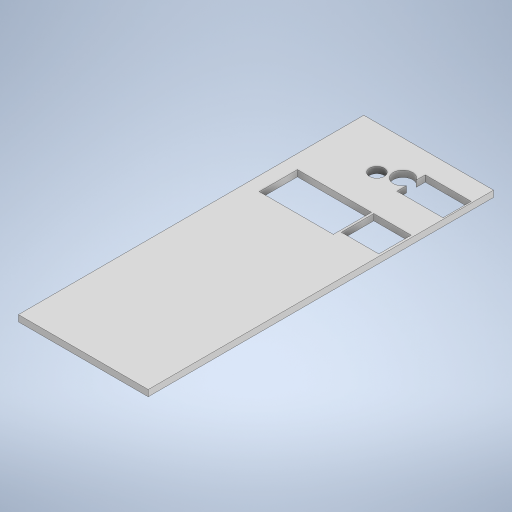
# Autodesk Inventor part: acrylicBackPanel
Saved by Autodesk Inventor 2023 (Build 270158000, 158)
## iProperties
Created: 2022-07-14
Part Number: acrylicBackPanel
Material: Generic
Document SubType Name: Modeling
Designer: Zain Ali
Density: 1 g/cm^3
Appearance: Default
Author: Zain Ali
Autodesk Inventor part; units mm, degrees
ref_plane "YZ Plane" through (0, 0, 0) normal (1, 0, 0) x (0, 1, 0)
ref_plane "XZ Plane" through (0, 0, 0) normal (0, 1, 0) x (-1, 0, 0)
ref_plane "XY Plane" through (0, 0, 0) normal (0, 0, 1) x (1, 0, 0)
sketch "Sketch1" plane through (0, 0, 0) normal (0, 1, 0) x (-1, 0, 0)
  line L0 (0, 0) -> (62, 0)
  line L1 (62, 0) -> (62, -165)
  line L2 (62, -165) -> (0, -165)
  line L3 (0, -165) -> (0, 0)
  dimension "d0" = 165
  dimension "d1" = 62
  constraints: 8 end point, 2 parallel, 1 horizontal, 1 perpendicular
  measures "d0" distance of L0.end L1.end
  measures "d1" distance of L1.end L2.end
extrude "Extrusion1" add sketch "Sketch1" along normal blind 3
sketch "Sketch2" plane through (0, 3, 0) normal (0, 1, 0) x (1, 0, 0)
  line L0 (-62, 165) -> (-62, 0)
  line L1 (3, 165) -> (-127, 165)
  circle A0 centre (-26.65, 148.375) radius 3.125
  line L2 (-18.9147, 111.2) -> (-1.0147, 111.2)
  line L3 (-1.0147, 111.2) -> (-1.0147, 126.7)
  line L4 (-1.0147, 126.7) -> (-18.9147, 126.7)
  line L5 (-18.9147, 126.7) -> (-18.9147, 111.2)
  line L6 (-17.6147, 112.2) -> (-2.3147, 112.2)
  line L7 (-7.804, 125.7) -> (-2.9647, 125.7)
  line L8 (-2.0147, 125.4) -> (-2.0147, 112.5)
  line L9 (-17.9147, 112.5) -> (-17.9147, 125.4)
  line L10 (-19.9657, 108.4) -> (-55.3657, 108.4)
  line L11 (-55.3657, 108.4) -> (-55.3657, 126.65)
  line L12 (-55.3657, 126.65) -> (-19.9657, 126.65)
  line L13 (-19.9657, 126.65) -> (-19.9657, 108.4)
  line L14 (-33.4157, 109.4) -> (-23.5157, 109.4)
  line L15 (-51.8157, 109.4) -> (-41.9157, 109.4)
  line L16 (-54.3657, 123.1) -> (-54.3657, 111.95)
  line L17 (-46.9157, 125.65) -> (-51.8157, 125.65)
  line L18 (-23.5157, 125.65) -> (-28.4157, 125.65)
  line L19 (-20.9657, 111.95) -> (-20.9657, 123.1)
  circle A1 centre (-26.65, 148.375) radius 4.625
  circle A2 centre (-35.25, 144.5) radius 3.5
  circle A3 centre (-35.25, 144.5) radius 2.5
  line L20 (-0.65, 141.5) -> (-22.65, 141.5)
  line L21 (-22.65, 141.5) -> (-22.65, 155)
  line L22 (-22.65, 155) -> (-0.65, 155)
  line L23 (-0.65, 155) -> (-0.65, 141.5)
  line L24 (-21.65, 142) -> (-1.65, 142)
  line L25 (-1.65, 142) -> (-1.65, 153)
  line L26 (-21.65, 153) -> (-1.65, 153)
  line L27 (-21.65, 142) -> (-21.65, 153)
  line L28 (0, 165) -> (-62, 165) projected
  line L29 (-62, 165) -> (-62, 0) projected
  point P0 (-35.25, 147)
  point P1 (-21.65, 147.5)
  point P2 (-22.65, 150.6968)
  point P3 (-22.65, 146.0532)
  dimension "d4" = 1
  dimension "d5" = 1
  dimension "d6" = 1
  dimension "d7" = 1
  dimension "d8" = 1
  dimension "d9" = 1
  dimension "d10" = 1
  dimension "d11" = 1
  dimension "d12" = 1.5
  dimension "d13" = 1
  dimension "d14" = 0.5
  dimension "d15" = 2
  dimension "d16" = 1
  dimension "d17" = 1
  dimension "d18" = 9.25
  dimension "d19" = 7
  dimension "d20" = 39.3
  dimension "d21" = 53.8
  dimension "d22" = 10
  dimension "d23" = 23.5
  dimension "d24" = 39.35
  dimension "d25" = 55.6
  dimension "d26" = 39.35
  dimension "d27" = 55.6
  dimension "d28" = 0.3647
  dimension "d29" = 17.2647
  dimension "d30" = 19.3157
  dimension "d31" = 21
  dimension "d32" = 53.7157
  dimension "d33" = 61.35
  dimension "d36" = 3.65
  dimension "d37" = 39.6
  dimension "d38" = 52.5
  dimension "d39" = 1.6647
  dimension "d40" = 2.3147
  dimension "d41" = 7.154
  dimension "d42" = 16.9647
  dimension "d43" = 39.6
  dimension "d44" = 52.5
  dimension "d45" = 41.9
  dimension "d46" = 53.05
  dimension "d47" = 22.8657
  dimension "d48" = 22.8657
  dimension "d49" = 26
  dimension "d50" = 27.7657
  dimension "d51" = 32.7657
  dimension "d52" = 18
  dimension "d53" = 34.6
  dimension "d54" = 34.6
  dimension "d55" = 41.2657
  dimension "d56" = 46.2657
  dimension "d57" = 51.1657
  dimension "d58" = 51.1657
  dimension "d59" = 41.9
  dimension "d60" = 53.05
  dimension "d61" = 0
  dimension "d62" = 165
  dimension "d63" = 126.35
  constraints: 56 end point, 11 parallel, 4 horizontal, 3 centre point, 3 perpendicular, 2 coincident, 2 collinear, 1 midpoint, 1 tangent, 1 vertical alignment, 1 other
  measures "d4" distance between parallel lines of L2 L6
  measures "d5" distance between parallel lines of L5 L9
  measures "d6" distance between parallel lines of L4 L7
  measures "d7" distance between parallel lines of L3 L8
  measures "d8" distance between parallel lines of L18 L12
  measures "d9" distance between parallel lines of L13 L19
  measures "d10" distance between parallel lines of L10 L14
  measures "d11" distance between parallel lines of L11 L16
  measures "d12" radial gap between concentric circles of A1 A0
  measures "d14" distance between parallel lines of L20 L24
  measures "d15" distance between parallel lines of L22 L26
  measures "d16" distance between parallel lines of L25 L23
  measures "d17" distance from line of point (-21.65, 147.5) L21
  measures "d18" diameter of A1
  measures "d19" diameter of A2
  measures "d20" distance between parallel lines of L1 L7
  measures "d21" distance between parallel lines of L1 L2
  measures "d22" distance between parallel lines of L1 L22
  measures "d23" distance between parallel lines of L1 L20
  measures "d24" distance between parallel lines of L1 L18
  measures "d25" distance between parallel lines of L1 L14
  measures "d26" distance between parallel lines of L1 L17
  measures "d27" distance between parallel lines of L1 L15
  measures "d28" distance between parallel lines of L23 L3
  measures "d29" distance between parallel lines of L9 L23
  measures "d30" distance between parallel lines of L23 L13
  measures "d31" distance between parallel lines of L23 L27
  measures "d32" distance between parallel lines of L16 L23
  measures "d33" distance between parallel lines of L23 L0
  measures "d36" distance from line of L1.start L23
  measures "d37" distance from line of L8.start L1
  measures "d38" distance from line of L8.end L1
  measures "d39" distance from line of L6.end L23
  measures "d40" distance from line of L7.end L23
  measures "d41" distance from line of L7.start L23
  measures "d42" distance from line of L6.start L23
  measures "d43" distance from line of L9.end L1
  measures "d44" distance from line of L9.start L1
  measures "d45" distance from line of L19.end L1
  measures "d46" distance from line of L19.start L1
  measures "d47" distance from line of L18.start L23
  measures "d48" distance from line of L14.end L23
  measures "d49" distance from line of A0.centre L23
  measures "d50" distance from line of L18.end L23
  measures "d51" distance from line of L14.start L23
  measures "d52" distance from line of point (-35.25, 147) L1
  measures "d53" distance from line of point (-35.25, 147) L23
  measures "d54" distance from line of point (-35.25, 144.5) L23
  measures "d55" distance from line of L15.end L23
  measures "d56" distance from line of L17.start L23
  measures "d57" distance from line of L17.end L23
  measures "d58" distance from line of L15.start L23
  measures "d59" distance from line of L16.start L1
  measures "d60" distance from line of L16.end L1
  measures "d61" distance from line of L0.start L1
  measures "d62" distance from line of L0.end L1
  measures "d63" distance from line of L1.end L23
extrude "Extrusion2" cut sketch "Sketch2" against normal through all contours A0 | L5 L4 L3 L2 | L10 L11 L12 L13 | A1 L21 | A1 L21 L22 L23 L20 | L21 A1 | A2 | A3 | L27 L26 L25 L24
body "Solid1"
